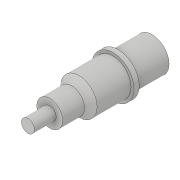
# Autodesk Inventor part: BC501A _Organic_scintillator_module
Saved by Autodesk Inventor 2019 (Build 230136000, 136)
## iProperties
Created: 2017-06-01
Part Number: BC501A _Organic_scintillator_module
Material: Generic
Document SubType Name: Modeling
Designer: Junsong
Density: 1 g/cm^3
Appearance: Default
Author: Junsong
Autodesk Inventor part; units mm, degrees
ref_plane "YZ Plane" through (0, 0, 0) normal (1, 0, 0) x (0, 1, 0)
ref_plane "XZ Plane" through (0, 0, 0) normal (0, 1, 0) x (-1, 0, 0)
sketch "Sketch1" plane through (0, 0, 0) normal (0, 0, 1) x (1, 0, 0)
  circle A0 centre (0, 0) radius 66.675
  dimension "d0" = 133.35
  constraints: 1 centre point, 1 coincident
  measures "d0" diameter of A0
extrude "Extrusion1" add sketch "Sketch1" along normal blind 133.35
sketch "Sketch2" plane through (0, 0, 133.35) normal (0, 0, 1) x (1, 0, 0)
  circle A0 centre (0, 0) radius 82.55
  dimension "d3" = 165.1
  constraints: 1 centre point, 1 coincident
  measures "d3" diameter of A0
extrude "Extrusion2" add sketch "Sketch2" along normal blind 20.6375
sketch "Sketch3" plane through (0, 0, 153.9875) normal (0, 0, 1) x (1, 0, 0)
  circle A0 centre (0, 0) radius 71.4375
  dimension "d6" = 142.875
  constraints: 1 centre point, 1 coincident
  measures "d6" diameter of A0
extrude "Extrusion3" add sketch "Sketch3" along normal blind 133.35
sketch "Sketch4" plane through (0, 0, 287.3375) normal (0, 0, 1) x (1, 0, 0)
  circle A0 centre (0, 0) radius 50.8
  dimension "d9" = 101.6
  constraints: 1 centre point, 1 coincident
  measures "d9" diameter of A0
extrude "Extrusion4" add sketch "Sketch4" along normal blind 114.3
sketch "Sketch5" plane through (0, 0, 401.6375) normal (0, 0, 1) x (1, 0, 0)
  circle A0 centre (0, 0) radius 25.4
  dimension "d12" = 50.8
  constraints: 1 centre point, 1 coincident
  measures "d12" diameter of A0
extrude "Extrusion5" add sketch "Sketch5" along normal blind 85.725
ref_plane "Work Plane1" through (0, 0, 487.3625) normal (0, 1, 0) x (0, 0, 1)
sketch "Sketch6" plane through (0, 0, 487.3625) normal (0, 1, 0) x (0, 0, 1)
  line L0 (-200.025, -71.4375) -> (-200.025, 71.4375) projected
  line L1 (-171.45, 50.8) -> (-200.025, 71.4375)
  line L2 (-85.725, -50.8) -> (-85.725, 50.8) projected
  line L3 (-85.725, 50.8) -> (-200.025, 50.8)
  line L4 (-200.025, 71.4375) -> (-200.025, 50.8)
  line L5 (-584.835, 0) -> (97.4725, 0) projected
  point P0 (-487.3625, 0)
  dimension "d21" = 28.575
  constraints: 6 end point, 2 point on line, 1 collinear, 1 perpendicular
  measures "d21" distance of L3.end L1.start
revolve "Revolution1" add sketch "Sketch6" angle 360 about axis through (0, 0, 487.3625) along (0, 0, 1) contours L0 L1 L3
body "Solid1"
